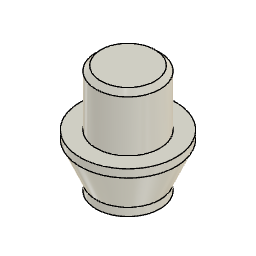
HANDLE_BUTTON v2 (Autodesk Fusion 360 design; units mm, degrees)
Autodesk Fusion 360 part; units mm, degrees
sketch "Schizzo1" plane through (0, 0, 0) normal (1, 0, 0) x (0, 1, 0)
  line L0 (0, 0) -> (0, 13.6)
  line L1 (0, 13.6) -> (4, 13.6)
  line L2 (4, 13.6) -> (4, 6.6)
  line L3 (4, 6.6) -> (6, 6.6)
  line L4 (6, 6.6) -> (6, 5.6)
  line L5 (6, 5.6) -> (4, 1)
  line L6 (4, 1) -> (4, 0)
  line L7 (4, 0) -> (0, 0)
  line L8 (0, 0) -> (0, -9.2) construction
  line L9 (0, -9.2) -> (10, -9.2) construction
  line L10 (0, -4) -> (10, -4) construction
  line L11 (0, 6.8) -> (10, 6.8) construction
  dimension "d1" = 8
  dimension "d2" = 8
  dimension "d3" = 7
  dimension "d4" = 10.8
  dimension "d5" = 16
  dimension "d6" = 0.2
  dimension "d7" = 10
  dimension "d8" = 2
  dimension "d10" = 4
  dimension "d11" = 1
  dimension "d12" = 1
  constraint coincident L0.start L7.end
  constraint vertical L0
  constraint perpendicular L0 L1
  constraint perpendicular L1 L2
  constraint perpendicular L0 L3
  constraint perpendicular L3 L4
  constraint perpendicular L3 L6
  constraint perpendicular L6 L7
  constraint perpendicular L7 L8
  constraint perpendicular L8 L9
  constraint coincident L8 L10.start
  constraint perpendicular L8 L10
  constraint coincident L8 L11.start
  constraint perpendicular L8 L11
  constraint equal L9 L10
  constraint equal L10 L11
  measures "d3" distance of L1 L3
  measures "d4" distance of L10 L11
  measures "d5" distance of L9 L11
  measures "d6" distance of L3 L11
  measures "d7" distance of L8.end L9.end
  measures "d8" distance of L2.end L3.end
  measures "d10" distance of L7 L10
  measures "d11" distance of L3.end L4.end
  measures "d12" distance of L5.end L6.end
revolve "Rivoluzione1" add sketch "Schizzo1" angle 360 about axis through (0, 0, 0) along (0, 0, 1)
chamfer "Smusso1" distance 0.6 angle 45 1 edges at (-3.7293, 1.4465, 13.6)
component "Component" placed x (1, 0, 0) y (0, 1, 0) z (0, 0, 1) at (0, 0, 0)
